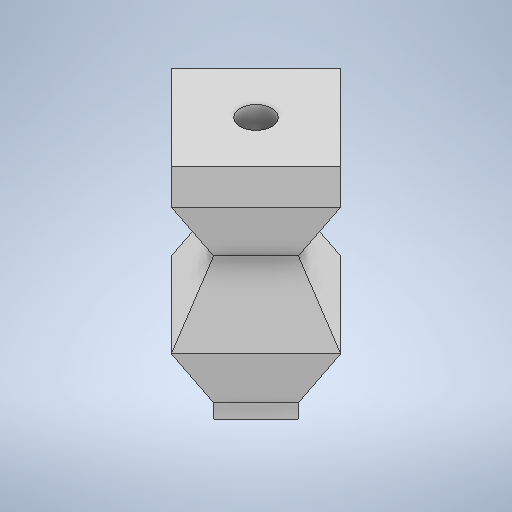
# Autodesk Inventor part: n_4
Saved by Autodesk Inventor 2025.1 (Build 291241000, 241)
## iProperties
Created: 2024-08-14
Part Number: n_4
Material: 일반
Document SubType Name: Modeling
Designer: 82103
Density: 1 g/cm^3
Appearance: 기본값
Author: 82103
Autodesk Inventor part; units mm, degrees
ref_plane "YZ Plane" through (0, 0, 0) normal (1, 0, 0) x (0, 1, 0)
ref_plane "XY Plane" through (0, 0, 0) normal (0, 0, 1) x (1, 0, 0)
sketch "스케치1" plane through (0, 0, 0) normal (0, 1, 0) x (-1, 0, 0)
  line L0 (12, 0) -> (0, -12)
  line L1 (0, -12) -> (-12, 0)
  line L2 (-12, 0) -> (0, 12)
  line L3 (0, 12) -> (12, 0)
  circle A0 centre (0, 0) radius 12 construction
  dimension "d0" = 24
  constraints: 8 end point, 2 coincident, 1 horizontal alignment, 1 vertical alignment, 11 other
ref_plane "작업 평면1" through (0, 9, 0) normal (0, 1, 0) x (-1, 0, 0)
sketch "스케치2" plane through (0, 9, 0) normal (0, 1, 0) x (-1, 0, 0)
  line L0 (6, 0) -> (0, -6)
  line L1 (0, -6) -> (-6, 0)
  line L2 (-6, 0) -> (0, 6)
  line L3 (0, 6) -> (6, 0)
  circle A0 centre (0, 0) radius 6 construction
  dimension "d2" = 12
  constraints: 8 end point, 2 coincident, 1 horizontal alignment, 1 vertical alignment, 11 other
loft "로프트1" add profiles "스케치2", "스케치1"
ref_plane "작업 평면2" through (0, 0, 0) normal (0, 1, 0) x (-1, 0, 0)
mirror "미러1" about plane through (0, 9, 0) normal (0, 1, 0) of "로프트1"
mirror "미러2" about plane through (0, 0, 0) normal (0, 1, 0) of "로프트1"
shell "쉘1" thickness 0.5 removed faces 0 ; own thickness 2 on faces at (-5.5, -1.5, -5.5) (5.5, -1.5, 5.5) (-5.5, -1.5, 5.5) (5.5, -1.5, -5.5) (-5.5, 16.5, -5.5) (5.5, 16.5, -5.5) (5.5, 16.5, 5.5) (-5.5, 16.5, 5.5)
sketch "스케치3" plane through (0, -9, -6) normal (0, -1, 0) x (0.7071068, 0, 0.7071068)
  line L0 (0, 8.4853) -> (0, 0) projected
  line L1 (0, 0) -> (8.4853, 0) projected
  line L2 (8.4853, 0) -> (8.4853, 8.4853) projected
  line L3 (8.4853, 8.4853) -> (0, 8.4853) projected
  point P0 (4.2426, 4.2426)
extrude "돌출1" add sketch "스케치3" along normal blind 2
sketch "스케치4" plane through (-12, 18, 0) normal (0, 1, 0) x (0.7071068, 0, 0.7071068)
  line L0 (0, 0) -> (0, 16.9706) projected
  line L1 (16.9706, 0) -> (0, 0) projected
  line L2 (16.9706, 16.9706) -> (16.9706, 0) projected
  line L3 (0, 16.9706) -> (16.9706, 16.9706) projected
  point P0 (8.4853, 8.4853)
extrude "돌출2" add sketch "스케치4" along normal blind 5
sketch "스케치5" plane through (-12, 23, 0) normal (0, 1, 0) x (0.7071068, 0, -0.7071068)
  circle A0 centre (8.4853, -8.4853) radius 2.25
  dimension "d14" = 4.5
  constraints: 1 centre point, 1 coincident
  measures "d14" diameter of A0
extrude "돌출3" cut sketch "스케치5" against normal blind 5.5
